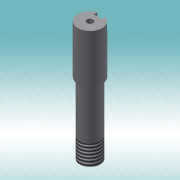
# Autodesk Inventor part: 回転アーム付き計測輪シャフト
Saved by Autodesk Inventor 2015 (Build 190159000, 159)
## iProperties
Created: 2016-04-01
Part Number: 回転アーム付き計測輪シャフト
Material: 一般
Document SubType Name: Modeling
Designer: buzztaka
Density: 1 g/cm^3
Appearance: 既定
Author: buzztaka
Autodesk Inventor part; units mm, degrees
ref_plane "YZ Plane" through (0, 0, 0) normal (1, 0, 0) x (0, 1, 0)
ref_plane "XZ Plane" through (0, 0, 0) normal (0, 1, 0) x (-1, 0, 0)
sketch "スケッチ1" plane through (0, 0, 0) normal (0, 0, 1) x (1, 0, 0)
  point P0 (0, 0)
sketch "スケッチ2" plane through (0, 0, 0) normal (0, 0, 1) x (1, 0, 0)
  circle A0 centre (0, 0) radius 5
  dimension "d0" = 10
  constraints: 1 centre point, 1 coincident
  measures "d0" diameter of A0
extrude "押し出し1" add sketch "スケッチ2" along normal blind 35
thread "ねじ1" size "M10x1.5" class "6g" standard "ANSI Metric M Profile" length 10
sketch "スケッチ3" plane through (0, 0, 35) normal (0, 0, 1) x (1, 0, 0)
  point P0 (0, 0)
sketch "スケッチ4" plane through (0, 0, 35) normal (0, 0, 1) x (1, 0, 0)
  circle A0 centre (0, 0) radius 6
  dimension "d5" = 12
  constraints: 1 centre point, 1 coincident
  measures "d5" diameter of A0
extrude "押し出し2" add sketch "スケッチ4" along normal blind 23.85
sketch "スケッチ5" plane through (0, 0, 58.85) normal (0, 0, 1) x (1, 0, 0)
  line L0 (0, 0) -> (0, 6)
  circle A0 centre (0, 0) radius 6 projected
  constraints: 2 end point, 1 vertical alignment, 1 other
ref_plane "作業平面1" through (0, 6, 58.85) normal (0, 1, 0) x (-1, 0, 0)
sketch "スケッチ6" plane through (0, 6, 58.85) normal (0, 1, 0) x (-1, 0, 0)
  line L0 (6, 0) -> (-6, 0) projected
  line L1 (-2, 0) -> (2, 0)
  line L2 (2, 0) -> (2, -13)
  line L3 (-2, -13) -> (-2, 0)
  arc A0 (-2, -13) -> (2, -13) centre (0, -13) ccw
  point P0 (0, -58.85)
  point P1 (0, 0)
  dimension "d8" = 2
  dimension "d9" = 2
  dimension "d12" = 4
  constraints: 6 end point, 2 point on circle, 2 point on line, 1 centre point, 1 horizontal, 1 midpoint, 1 parallel, 1 perpendicular
  measures "d8" distance of point (0, 0) point (2, 0)
  measures "d9" distance of L1.start point (0, 0)
  measures "d12" diameter of A0
extrude "押し出し3" cut sketch "スケッチ6" against normal blind 2.157
sketch "スケッチ7" plane through (0, 0, 58.85) normal (0, 0, 1) x (1, 0, 0)
  point P0 (0, 0)
  point P1 (0, 0)
  constraints: 1 coincident
hole "穴1" at (0, 0, 58.85) direction (0, 0, -1) diameter 3 depth 8 tip angle 118
thread "ねじ2" size "M3x0.5" class "6H" standard "ANSI Metric M Profile" full length
